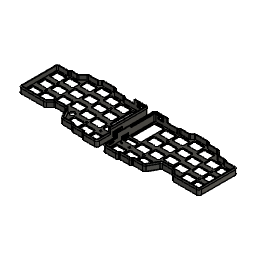
mriya-bumper-mjf-v1.14 (Autodesk Fusion 360 design; units mm, degrees)
Autodesk Fusion 360 part; units mm, degrees
(part 1 of 2)
sketch "mriya-bumper-mjf" plane through (0, 0, 0) normal (0, 0, 1) x (1, 0, 0)
  line L0 (-101.0213, 15.6719) -> (-94.7787, 21.9145) construction
  line L1 (-26.4858, 1.079) -> (-27.6142, 2.2074) construction
  line L2 (-138.1, 14.7932) -> (-103.1426, 14.7932) construction
  line L3 (-44.0716, 2.7932) -> (-29.0284, 2.7932) construction
  line L4 (-8.6, 0.4932) -> (-25.0716, 0.4932) construction
  line L5 (-64.4741, 6.1094) -> (-72.7517, 20.7608) construction
  line L6 (-45.4858, 3.379) -> (-46.6142, 4.5074) construction
  line L7 (-122.6142, 71.579) -> (-121.4858, 72.7074) construction
  line L8 (-101.0716, 81.2932) -> (-87.2284, 81.2932) construction
  line L9 (-138.1, 70.9932) -> (-124.0284, 70.9932) construction
  line L10 (-92.6574, 22.7932) -> (-76.2344, 22.7932) construction
  line L11 (-48.0284, 5.0932) -> (-62.7328, 5.0932) construction
  line L12 (-82.0716, 84.7932) -> (-64.7284, 84.7932) construction
  line L13 (-58.5716, 80.2932) -> (-45.7284, 80.2932) construction
  line L14 (-24.8, 19.4932) -> (-7.1, 19.4932) construction
  line L15 (-25.6, 20.2932) -> (-25.6, 77.9932) construction
  line L16 (-83.4858, 84.2074) -> (-85.8142, 81.879) construction
  line L17 (-63.3142, 84.2074) -> (-59.9858, 80.879) construction
  line L18 (-139.6, 69.4932) -> (-139.6, 16.2932) construction
  line L19 (-43.1858, 78.579) -> (-44.3142, 79.7074) construction
  line L20 (-99.4, 40.3932) -> (-99.4, 27.9932) construction
  line L21 (-98.6, 41.1932) -> (-86.2, 41.1932) construction
  line L22 (-98.6, 27.1932) -> (-86.2, 27.1932) construction
  line L23 (-85.4, 40.3932) -> (-85.4, 27.9932) construction
  line L24 (-42.4, 56.0932) -> (-42.4, 43.6932) construction
  line L25 (-41.6, 56.8932) -> (-29.2, 56.8932) construction
  line L26 (-41.6, 42.8932) -> (-29.2, 42.8932) construction
  line L27 (-28.4, 56.0932) -> (-28.4, 43.6932) construction
  line L28 (-61.4, 58.3932) -> (-61.4, 45.9932) construction
  line L29 (-60.6, 59.1932) -> (-48.2, 59.1932) construction
  line L30 (-60.6, 45.1932) -> (-48.2, 45.1932) construction
  line L31 (-47.4, 58.3932) -> (-47.4, 45.9932) construction
  line L32 (-137.4, 68.0932) -> (-137.4, 55.6932) construction
  line L33 (-136.6, 68.8932) -> (-124.2, 68.8932) construction
  line L34 (-136.6, 54.8932) -> (-124.2, 54.8932) construction
  line L35 (-123.4, 68.0932) -> (-123.4, 55.6932) construction
  line L36 (-61.4, 39.3932) -> (-61.4, 26.9932) construction
  line L37 (-60.6, 40.1932) -> (-48.2, 40.1932) construction
  line L38 (-60.6, 26.1932) -> (-48.2, 26.1932) construction
  line L39 (-47.4, 39.3932) -> (-47.4, 26.9932) construction
  line L40 (-42.4, 18.0932) -> (-42.4, 5.6932) construction
  line L41 (-41.6, 18.8932) -> (-29.2, 18.8932) construction
  line L42 (-41.6, 4.8932) -> (-29.2, 4.8932) construction
  line L43 (-28.4, 18.0932) -> (-28.4, 5.6932) construction
  line L44 (-23.4, 15.7932) -> (-23.4, 3.3932) construction
  line L45 (-22.6, 16.5932) -> (-10.2, 16.5932) construction
  line L46 (-22.6, 2.5932) -> (-10.2, 2.5932) construction
  line L47 (-9.4, 15.7932) -> (-9.4, 3.3932) construction
  line L48 (-137.4, 49.0932) -> (-137.4, 36.6932) construction
  line L49 (-136.6, 49.8932) -> (-124.2, 49.8932) construction
  line L50 (-136.6, 35.8932) -> (-124.2, 35.8932) construction
  line L51 (-123.4, 49.0932) -> (-123.4, 36.6932) construction
  line L52 (-118.4, 51.3932) -> (-118.4, 38.9932) construction
  line L53 (-117.6, 52.1932) -> (-105.2, 52.1932) construction
  line L54 (-117.6, 38.1932) -> (-105.2, 38.1932) construction
  line L55 (-104.4, 51.3932) -> (-104.4, 38.9932) construction
  line L56 (-137.4, 30.0932) -> (-137.4, 17.6932) construction
  line L57 (-136.6, 30.8932) -> (-124.2, 30.8932) construction
  line L58 (-136.6, 16.8932) -> (-124.2, 16.8932) construction
  line L59 (-123.4, 30.0932) -> (-123.4, 17.6932) construction
  line L60 (-61.4, 20.3932) -> (-61.4, 7.9932) construction
  line L61 (-60.6, 21.1932) -> (-48.2, 21.1932) construction
  line L62 (-60.6, 7.1932) -> (-48.2, 7.1932) construction
  line L63 (-47.4, 20.3932) -> (-47.4, 7.9932) construction
  line L64 (-80.4, 43.8932) -> (-80.4, 31.4932) construction
  line L65 (-79.6, 44.6932) -> (-67.2, 44.6932) construction
  line L66 (-79.6, 30.6932) -> (-67.2, 30.6932) construction
  line L67 (-66.4, 43.8932) -> (-66.4, 31.4932) construction
  line L68 (-80.4, 81.8932) -> (-80.4, 69.4932) construction
  line L69 (-79.6, 82.6932) -> (-67.2, 82.6932) construction
  line L70 (-79.6, 68.6932) -> (-67.2, 68.6932) construction
  line L71 (-66.4, 81.8932) -> (-66.4, 69.4932) construction
  line L72 (-42.4, 37.0932) -> (-42.4, 24.6932) construction
  line L73 (-41.6, 37.8932) -> (-29.2, 37.8932) construction
  line L74 (-41.6, 23.8932) -> (-29.2, 23.8932) construction
  line L75 (-28.4, 37.0932) -> (-28.4, 24.6932) construction
  line L76 (-118.4, 32.3932) -> (-118.4, 19.9932) construction
  line L77 (-117.6, 33.1932) -> (-105.2, 33.1932) construction
  line L78 (-117.6, 19.1932) -> (-105.2, 19.1932) construction
  line L79 (-104.4, 32.3932) -> (-104.4, 19.9932) construction
  line L80 (-61.4, 77.3932) -> (-61.4, 64.9932) construction
  line L81 (-60.6, 78.1932) -> (-48.2, 78.1932) construction
  line L82 (-60.6, 64.1932) -> (-48.2, 64.1932) construction
  line L83 (-47.4, 77.3932) -> (-47.4, 64.9932) construction
  line L84 (-42.4, 75.0932) -> (-42.4, 62.6932) construction
  line L85 (-41.6, 75.8932) -> (-29.2, 75.8932) construction
  line L86 (-41.6, 61.8932) -> (-29.2, 61.8932) construction
  line L87 (-28.4, 75.0932) -> (-28.4, 62.6932) construction
  line L88 (-118.4, 70.3932) -> (-118.4, 57.9932) construction
  line L89 (-117.6, 71.1932) -> (-105.2, 71.1932) construction
  line L90 (-117.6, 57.1932) -> (-105.2, 57.1932) construction
  line L91 (-104.4, 70.3932) -> (-104.4, 57.9932) construction
  line L92 (-99.4, 59.3932) -> (-99.4, 46.9932) construction
  line L93 (-98.6, 60.1932) -> (-86.2, 60.1932) construction
  line L94 (-98.6, 46.1932) -> (-86.2, 46.1932) construction
  line L95 (-85.4, 59.3932) -> (-85.4, 46.9932) construction
  line L96 (-80.4, 62.8932) -> (-80.4, 50.4932) construction
  line L97 (-79.6, 63.6932) -> (-67.2, 63.6932) construction
  line L98 (-79.6, 49.6932) -> (-67.2, 49.6932) construction
  line L99 (-66.4, 62.8932) -> (-66.4, 50.4932) construction
  line L100 (-99.4, 78.3932) -> (-99.4, 65.9932) construction
  line L101 (-98.6, 79.1932) -> (-86.2, 79.1932) construction
  line L102 (-98.6, 65.1932) -> (-86.2, 65.1932) construction
  line L103 (-85.4, 78.3932) -> (-85.4, 65.9932) construction
  circle A0 centre (-120.9, 53.5432) radius 1.7
  circle A1 centre (-120.9, 34.5432) radius 1.7
  circle A2 centre (-68.5, 23.5932) radius 4
  circle A3 centre (-44.9, 22.5432) radius 1.7
  circle A4 centre (-44.9, 60.5432) radius 1.7
  arc A5 (-43.1858, 78.579) -> (-41.7716, 77.9932) centre (-41.7716, 79.9932) ccw construction
  arc A6 (-44.3142, 79.7074) -> (-45.7284, 80.2932) centre (-45.7285, 78.2931) ccw construction
  arc A7 (-59.9858, 80.879) -> (-58.5716, 80.2932) centre (-58.5716, 82.2931) ccw construction
  arc A8 (-63.3142, 84.2074) -> (-64.7284, 84.7932) centre (-64.7285, 82.7931) ccw construction
  arc A9 (-82.0716, 84.7932) -> (-83.4858, 84.2074) centre (-82.0716, 82.7933) ccw construction
  arc A10 (-87.2284, 81.2932) -> (-85.8142, 81.879) centre (-87.2284, 83.2932) ccw construction
  arc A11 (-101.0716, 81.2932) -> (-102.4858, 80.7074) centre (-101.0716, 79.2933) ccw construction
  arc A12 (-120.0716, 73.2932) -> (-121.4858, 72.7074) centre (-120.0716, 71.2933) ccw construction
  arc A13 (-124.0284, 70.9932) -> (-122.6142, 71.579) centre (-124.0284, 72.9932) ccw construction
  arc A14 (-138.1, 70.9932) -> (-139.6, 69.4932) centre (-138.1, 69.4932) ccw construction
  arc A15 (-139.6, 16.2932) -> (-138.1, 14.7932) centre (-138.1, 16.2932) ccw construction
  arc A16 (-103.1426, 14.7932) -> (-101.0213, 15.6719) centre (-103.1426, 17.7931) ccw construction
  arc A17 (-92.6574, 22.7932) -> (-94.7787, 21.9145) centre (-92.6573, 19.7931) ccw construction
  arc A18 (-72.7517, 20.7608) -> (-76.2344, 22.7932) centre (-76.2344, 18.793) ccw construction
  arc A19 (-64.4741, 6.1094) -> (-62.7328, 5.0932) centre (-62.7328, 7.0932) ccw construction
  arc A20 (-46.6142, 4.5074) -> (-48.0284, 5.0932) centre (-48.0284, 3.0933) ccw construction
  arc A21 (-45.4858, 3.379) -> (-44.0716, 2.7932) centre (-44.0715, 4.7933) ccw construction
  arc A22 (-27.6142, 2.2074) -> (-29.0284, 2.7932) centre (-29.0284, 0.7933) ccw construction
  arc A23 (-26.4858, 1.079) -> (-25.0716, 0.4932) centre (-25.0715, 2.4933) ccw construction
  arc A24 (-8.6, 0.4932) -> (-7.1, 1.9932) centre (-8.6, 1.9932) ccw construction
  line L104 (-7.1, 1.9932) -> (-7.1, 76.4932) construction
  line L105 (-41.7716, 77.9932) -> (-8.6, 77.9932) construction
  arc A25 (-7.1, 76.4932) -> (-8.6, 77.9932) centre (-8.6, 76.4932) ccw construction
  arc A26 (-136.6, 68.8932) -> (-137.4, 68.0932) centre (-136.6, 68.0932) ccw construction
  arc A27 (-123.4, 68.0932) -> (-124.2, 68.8932) centre (-124.2, 68.0932) ccw construction
  arc A28 (-124.2, 54.8932) -> (-123.4, 55.6932) centre (-124.2, 55.6932) ccw construction
  arc A29 (-137.4, 55.6932) -> (-136.6, 54.8932) centre (-136.6, 55.6932) ccw construction
  arc A30 (-136.6, 49.8932) -> (-137.4, 49.0932) centre (-136.6, 49.0932) ccw construction
  arc A31 (-123.4, 49.0932) -> (-124.2, 49.8932) centre (-124.2, 49.0932) ccw construction
  arc A32 (-124.2, 35.8932) -> (-123.4, 36.6932) centre (-124.2, 36.6932) ccw construction
  arc A33 (-137.4, 36.6932) -> (-136.6, 35.8932) centre (-136.6, 36.6932) ccw construction
  arc A34 (-136.6, 30.8932) -> (-137.4, 30.0932) centre (-136.6, 30.0932) ccw construction
  arc A35 (-123.4, 30.0932) -> (-124.2, 30.8932) centre (-124.2, 30.0932) ccw construction
  arc A36 (-124.2, 16.8932) -> (-123.4, 17.6932) centre (-124.2, 17.6932) ccw construction
  arc A37 (-137.4, 17.6932) -> (-136.6, 16.8932) centre (-136.6, 17.6932) ccw construction
  arc A38 (-118.4, 19.9932) -> (-117.6, 19.1932) centre (-117.6, 19.9932) ccw construction
  arc A39 (-105.2, 19.1932) -> (-104.4, 19.9932) centre (-105.2, 19.9932) ccw construction
  arc A40 (-104.4, 32.3932) -> (-105.2, 33.1932) centre (-105.2, 32.3932) ccw construction
  arc A41 (-117.6, 33.1932) -> (-118.4, 32.3932) centre (-117.6, 32.3932) ccw construction
  arc A42 (-105.2, 38.1932) -> (-104.4, 38.9932) centre (-105.2, 38.9932) ccw construction
  arc A43 (-118.4, 38.9932) -> (-117.6, 38.1932) centre (-117.6, 38.9932) ccw construction
  arc A44 (-117.6, 52.1932) -> (-118.4, 51.3932) centre (-117.6, 51.3932) ccw construction
  arc A45 (-104.4, 51.3932) -> (-105.2, 52.1932) centre (-105.2, 51.3932) ccw construction
  arc A46 (-118.4, 57.9932) -> (-117.6, 57.1932) centre (-117.6, 57.9932) ccw construction
  arc A47 (-105.2, 57.1932) -> (-104.4, 57.9932) centre (-105.2, 57.9932) ccw construction
  arc A48 (-104.4, 70.3932) -> (-105.2, 71.1932) centre (-105.2, 70.3932) ccw construction
  arc A49 (-117.6, 71.1932) -> (-118.4, 70.3932) centre (-117.6, 70.3932) ccw construction
  arc A50 (-98.6, 79.1932) -> (-99.4, 78.3932) centre (-98.6, 78.3932) ccw construction
  arc A51 (-85.4, 78.3932) -> (-86.2, 79.1932) centre (-86.2, 78.3932) ccw construction
  arc A52 (-86.2, 65.1932) -> (-85.4, 65.9932) centre (-86.2, 65.9932) ccw construction
  arc A53 (-99.4, 65.9932) -> (-98.6, 65.1932) centre (-98.6, 65.9932) ccw construction
  arc A54 (-98.6, 60.1932) -> (-99.4, 59.3932) centre (-98.6, 59.3932) ccw construction
  arc A55 (-85.4, 59.3932) -> (-86.2, 60.1932) centre (-86.2, 59.3932) ccw construction
  arc A56 (-86.2, 46.1932) -> (-85.4, 46.9932) centre (-86.2, 46.9932) ccw construction
  arc A57 (-99.4, 46.9932) -> (-98.6, 46.1932) centre (-98.6, 46.9932) ccw construction
  arc A58 (-98.6, 41.1932) -> (-99.4, 40.3932) centre (-98.6, 40.3932) ccw construction
  arc A59 (-99.4, 27.9932) -> (-98.6, 27.1932) centre (-98.6, 27.9932) ccw construction
  arc A60 (-86.2, 27.1932) -> (-85.4, 27.9932) centre (-86.2, 27.9932) ccw construction
  arc A61 (-85.4, 40.3932) -> (-86.2, 41.1932) centre (-86.2, 40.3932) ccw construction
  arc A62 (-80.4, 31.4932) -> (-79.6, 30.6932) centre (-79.6, 31.4932) ccw construction
  arc A63 (-79.6, 44.6932) -> (-80.4, 43.8932) centre (-79.6, 43.8932) ccw construction
  arc A64 (-66.4, 43.8932) -> (-67.2, 44.6932) centre (-67.2, 43.8932) ccw construction
  arc A65 (-67.2, 30.6932) -> (-66.4, 31.4932) centre (-67.2, 31.4932) ccw construction
  arc A66 (-67.2, 49.6932) -> (-66.4, 50.4932) centre (-67.2, 50.4932) ccw construction
  arc A67 (-80.4, 50.4932) -> (-79.6, 49.6932) centre (-79.6, 50.4932) ccw construction
  arc A68 (-79.6, 63.6932) -> (-80.4, 62.8932) centre (-79.6, 62.8932) ccw construction
  arc A69 (-66.4, 62.8932) -> (-67.2, 63.6932) centre (-67.2, 62.8932) ccw construction
  arc A70 (-67.2, 68.6932) -> (-66.4, 69.4932) centre (-67.2, 69.4932) ccw construction
  arc A71 (-80.4, 69.4932) -> (-79.6, 68.6932) centre (-79.6, 69.4932) ccw construction
  arc A72 (-79.6, 82.6932) -> (-80.4, 81.8932) centre (-79.6, 81.8932) ccw construction
  arc A73 (-66.4, 81.8932) -> (-67.2, 82.6932) centre (-67.2, 81.8932) ccw construction
  arc A74 (-60.6, 78.1932) -> (-61.4, 77.3932) centre (-60.6, 77.3932) ccw construction
  arc A75 (-61.4, 64.9932) -> (-60.6, 64.1932) centre (-60.6, 64.9932) ccw construction
  arc A76 (-48.2, 64.1932) -> (-47.4, 64.9932) centre (-48.2, 64.9932) ccw construction
  arc A77 (-47.4, 77.3932) -> (-48.2, 78.1932) centre (-48.2, 77.3932) ccw construction
  arc A78 (-47.4, 58.3932) -> (-48.2, 59.1932) centre (-48.2, 58.3932) ccw construction
  arc A79 (-60.6, 59.1932) -> (-61.4, 58.3932) centre (-60.6, 58.3932) ccw construction
  arc A80 (-61.4, 45.9932) -> (-60.6, 45.1932) centre (-60.6, 45.9932) ccw construction
  arc A81 (-48.2, 45.1932) -> (-47.4, 45.9932) centre (-48.2, 45.9932) ccw construction
  arc A82 (-47.4, 39.3932) -> (-48.2, 40.1932) centre (-48.2, 39.3932) ccw construction
  arc A83 (-60.6, 40.1932) -> (-61.4, 39.3932) centre (-60.6, 39.3932) ccw construction
  arc A84 (-61.4, 26.9932) -> (-60.6, 26.1932) centre (-60.6, 26.9932) ccw construction
  arc A85 (-48.2, 26.1932) -> (-47.4, 26.9932) centre (-48.2, 26.9932) ccw construction
  arc A86 (-47.4, 20.3932) -> (-48.2, 21.1932) centre (-48.2, 20.3932) ccw construction
  arc A87 (-60.6, 21.1932) -> (-61.4, 20.3932) centre (-60.6, 20.3932) ccw construction
  arc A88 (-61.4, 7.9932) -> (-60.6, 7.1932) centre (-60.6, 7.9932) ccw construction
  arc A89 (-48.2, 7.1932) -> (-47.4, 7.9932) centre (-48.2, 7.9932) ccw construction
  arc A90 (-42.4, 5.6932) -> (-41.6, 4.8932) centre (-41.6, 5.6932) ccw construction
  arc A91 (-29.2, 4.8932) -> (-28.4, 5.6932) centre (-29.2, 5.6932) ccw construction
  arc A92 (-28.4, 18.0932) -> (-29.2, 18.8932) centre (-29.2, 18.0932) ccw construction
  arc A93 (-41.6, 18.8932) -> (-42.4, 18.0932) centre (-41.6, 18.0932) ccw construction
  arc A94 (-23.4, 3.3932) -> (-22.6, 2.5932) centre (-22.6, 3.3932) ccw construction
  arc A95 (-10.2, 2.5932) -> (-9.4, 3.3932) centre (-10.2, 3.3932) ccw construction
  arc A96 (-9.4, 15.7932) -> (-10.2, 16.5932) centre (-10.2, 15.7932) ccw construction
  arc A97 (-22.6, 16.5932) -> (-23.4, 15.7932) centre (-22.6, 15.7932) ccw construction
  arc A98 (-29.2, 23.8932) -> (-28.4, 24.6932) centre (-29.2, 24.6932) ccw construction
  arc A99 (-42.4, 24.6932) -> (-41.6, 23.8932) centre (-41.6, 24.6932) ccw construction
  arc A100 (-41.6, 37.8932) -> (-42.4, 37.0932) centre (-41.6, 37.0932) ccw construction
  arc A101 (-28.4, 37.0932) -> (-29.2, 37.8932) centre (-29.2, 37.0932) ccw construction
  arc A102 (-29.2, 42.8932) -> (-28.4, 43.6932) centre (-29.2, 43.6932) ccw construction
  arc A103 (-42.4, 43.6932) -> (-41.6, 42.8932) centre (-41.6, 43.6932) ccw construction
  arc A104 (-41.6, 56.8932) -> (-42.4, 56.0932) centre (-41.6, 56.0932) ccw construction
  arc A105 (-28.4, 56.0932) -> (-29.2, 56.8932) centre (-29.2, 56.0932) ccw construction
  arc A106 (-29.2, 61.8932) -> (-28.4, 62.6932) centre (-29.2, 62.6932) ccw construction
  arc A107 (-42.4, 62.6932) -> (-41.6, 61.8932) centre (-41.6, 62.6932) ccw construction
  arc A108 (-41.6, 75.8932) -> (-42.4, 75.0932) centre (-41.6, 75.0932) ccw construction
  arc A109 (-28.4, 75.0932) -> (-29.2, 75.8932) centre (-29.2, 75.0932) ccw construction
  circle A110 centre (-22.6, 22.4932) radius 1.1
  circle A111 centre (-10.1, 22.4932) radius 1.1
  line L106 (-7, 19.2932) -> (-4.5, 19.2932)
  line L107 (-25.8, 78.0932) -> (-25.8, 80.5932)
  line L108 (-20.5, 77.4932) -> (-8.6, 77.4932)
  line L109 (-7.6, 40.5932) -> (-7.6, 76.4932)
  line L110 (-7.6, 12.9932) -> (-7.6, 6.1932)
  line L111 (-102.4858, 80.7074) -> (-109.0213, 74.1719) construction
  line L112 (-120.0716, 73.2932) -> (-111.1426, 73.2932) construction
  arc A112 (-111.1426, 73.2932) -> (-109.0213, 74.1719) centre (-111.1426, 76.2932) ccw construction
  arc A113 (-64.7284, 82.7932) -> (-64.7285, 82.7932) centre (-64.7285, 82.7931) ccw
  arc A114 (-45.7284, 78.2932) -> (-45.7285, 78.2932) centre (-45.7285, 78.2931) ccw
  arc A115 (-25.0716, 2.4932) -> (-25.0715, 2.4932) centre (-25.0715, 2.4933) ccw
  arc A116 (-44.0716, 4.7932) -> (-44.0715, 4.7932) centre (-44.0715, 4.7933) ccw
  line L113 (-138.9, 58.3932) -> (-138.9, 66.8932)
  line L114 (-136.9, 68.8932) -> (-123.9, 68.8932)
  arc A117 (-121.9, 66.8932) -> (-123.9, 68.8932) centre (-123.9, 66.8932) ccw
  arc A118 (-136.9, 68.8932) -> (-138.9, 66.8932) centre (-136.9, 66.8932) ccw
  line L115 (-104.9, 58.6932) -> (-117.9, 58.6932)
  line L116 (-119.9, 60.6932) -> (-119.9, 69.1932)
  arc A119 (-117.9, 71.1932) -> (-119.9, 69.1932) centre (-117.9, 69.1932) ccw
  line L117 (-117.9, 71.1932) -> (-104.9, 71.1932)
  arc A120 (-102.9, 69.1932) -> (-104.9, 71.1932) centre (-104.9, 69.1932) ccw
  line L118 (-102.9, 69.1932) -> (-102.9, 60.6932)
  line L119 (-85.9, 66.6932) -> (-98.9, 66.6932)
  line L120 (-100.9, 68.6932) -> (-100.9, 77.1932)
  arc A121 (-98.9, 79.1932) -> (-100.9, 77.1932) centre (-98.9, 77.1932) ccw
  line L121 (-98.9, 79.1932) -> (-85.9, 79.1932)
  arc A122 (-83.9, 77.1932) -> (-85.9, 79.1932) centre (-85.9, 77.1932) ccw
  line L122 (-83.9, 77.1932) -> (-83.9, 68.6932)
  line L123 (-66.9, 70.1932) -> (-79.9, 70.1932)
  line L124 (-81.9, 72.1932) -> (-81.9, 80.6932)
  arc A123 (-79.9, 82.6932) -> (-81.9, 80.6932) centre (-79.9, 80.6932) ccw
  line L125 (-79.9, 82.6932) -> (-66.9, 82.6932)
  arc A124 (-64.9, 80.6932) -> (-66.9, 82.6932) centre (-66.9, 80.6932) ccw
  line L126 (-64.9, 80.6932) -> (-64.9, 72.1932)
  line L127 (-47.9, 65.6932) -> (-60.9, 65.6932)
  line L128 (-62.9, 67.6932) -> (-62.9, 76.1932)
  arc A125 (-60.9, 78.1932) -> (-62.9, 76.1932) centre (-60.9, 76.1932) ccw
  line L129 (-60.9, 78.1932) -> (-47.9, 78.1932)
  arc A126 (-45.9, 76.1932) -> (-47.9, 78.1932) centre (-47.9, 76.1932) ccw
  line L130 (-45.9, 76.1932) -> (-45.9, 67.6932)
  line L131 (-43.9, 65.3932) -> (-43.9, 73.8932)
  arc A127 (-41.9, 75.8932) -> (-43.9, 73.8932) centre (-41.9, 73.8932) ccw
  line L132 (-41.9, 75.8932) -> (-28.9, 75.8932)
  arc A128 (-26.9, 73.8932) -> (-28.9, 75.8932) centre (-28.9, 73.8932) ccw
  line L133 (-26.9, 73.8932) -> (-26.9, 65.3932)
  arc A129 (-9.9, 26.8932) -> (-7.9, 28.8932) centre (-9.9, 28.8932) ccw
  line L134 (-9.9, 26.8932) -> (-22.9, 26.8932)
  arc A130 (-24.9, 28.8932) -> (-22.9, 26.8932) centre (-22.9, 28.8932) ccw
  arc A131 (-22.9, 75.8932) -> (-24.9, 73.8932) centre (-22.9, 73.8932) ccw
  arc A132 (-7.9, 73.8932) -> (-9.9, 75.8932) centre (-9.9, 73.8932) ccw
  line L135 (-28.9, 63.3932) -> (-41.9, 63.3932)
  line L136 (-121.9, 66.8932) -> (-121.9, 58.3932)
  line L137 (-123.9, 56.3932) -> (-136.9, 56.3932)
  line L138 (-122.6849, 71.6497) -> (-121.5565, 72.7781)
  arc A133 (-120.0716, 73.3932) -> (-121.5565, 72.7781) centre (-120.0716, 71.2933) ccw
  line L139 (-120.0716, 73.3932) -> (-111.1426, 73.3932)
  arc A134 (-111.1426, 73.3932) -> (-109.092, 74.2426) centre (-111.1426, 76.2932) ccw
  line L140 (-102.5565, 80.7781) -> (-109.092, 74.2426)
  arc A135 (-101.0716, 81.3932) -> (-102.5565, 80.7781) centre (-101.0716, 79.2933) ccw
  line L141 (-101.0716, 81.3932) -> (-87.2284, 81.3932)
  arc A136 (-87.2284, 81.3932) -> (-85.8849, 81.9497) centre (-87.2284, 83.2932) ccw
  line L142 (-83.5565, 84.2781) -> (-85.8849, 81.9497)
  arc A137 (-82.0716, 84.8932) -> (-83.5565, 84.2781) centre (-82.0716, 82.7933) ccw
  line L143 (-82.0716, 84.8932) -> (-64.7284, 84.8932)
  arc A138 (-63.2435, 84.2781) -> (-64.7284, 84.8932) centre (-64.7285, 82.7931) ccw
  line L144 (-63.2435, 84.2781) -> (-59.9151, 80.9497)
  arc A139 (-59.9151, 80.9497) -> (-58.5716, 80.3932) centre (-58.5716, 82.2931) ccw
  line L145 (-58.5716, 80.3932) -> (-45.7284, 80.3932)
  arc A140 (-44.2435, 79.7781) -> (-45.7284, 80.3932) centre (-45.7285, 78.2931) ccw
  line L146 (-43.1151, 78.6497) -> (-44.2435, 79.7781)
  arc A141 (-43.1151, 78.6497) -> (-41.7716, 78.0932) centre (-41.7716, 79.9932) ccw
  line L147 (-41.7716, 78.0932) -> (-8.6, 78.0932)
  arc A142 (-7, 76.4932) -> (-8.6, 78.0932) centre (-8.6, 76.4932) ccw
  line L148 (-7, 1.9932) -> (-7, 76.4932)
  arc A143 (-8.6, 0.3932) -> (-7, 1.9932) centre (-8.6, 1.9932) ccw
  line L149 (-8.6, 0.3932) -> (-25.0716, 0.3932)
  arc A144 (-26.5565, 1.0083) -> (-25.0716, 0.3932) centre (-25.0715, 2.4933) ccw
  line L150 (-26.5565, 1.0083) -> (-27.6849, 2.1367)
  arc A145 (-27.6849, 2.1367) -> (-29.0284, 2.6932) centre (-29.0284, 0.7933) ccw
  line L151 (-44.0716, 2.6932) -> (-29.0284, 2.6932)
  arc A146 (-45.5565, 3.3083) -> (-44.0716, 2.6932) centre (-44.0715, 4.7933) ccw
  line L152 (-45.5565, 3.3083) -> (-46.6849, 4.4367)
  arc A147 (-46.6849, 4.4367) -> (-48.0284, 4.9932) centre (-48.0284, 3.0933) ccw
  line L153 (-48.0284, 4.9932) -> (-62.7328, 4.9932)
  arc A148 (-64.5612, 6.0602) -> (-62.7328, 4.9932) centre (-62.7328, 7.0932) ccw
  line L154 (-64.5612, 6.0602) -> (-72.8388, 20.7116)
  arc A149 (-72.8388, 20.7116) -> (-76.2344, 22.6932) centre (-76.2344, 18.793) ccw
  line L155 (-92.6574, 22.6932) -> (-76.2344, 22.6932)
  arc A150 (-92.6574, 22.6932) -> (-94.708, 21.8438) centre (-92.6573, 19.7931) ccw
  line L156 (-100.9506, 15.6012) -> (-94.708, 21.8438)
  arc A151 (-103.1426, 14.6932) -> (-100.9506, 15.6012) centre (-103.1426, 17.7931) ccw
  line L157 (-138.1, 14.6932) -> (-103.1426, 14.6932)
  arc A152 (-139.7, 16.2932) -> (-138.1, 14.6932) centre (-138.1, 16.2932) ccw
  line L158 (-139.7, 69.4932) -> (-139.7, 16.2932)
  arc A153 (-138.1, 71.0932) -> (-139.7, 69.4932) centre (-138.1, 69.4932) ccw
  line L159 (-138.1, 71.0932) -> (-124.0284, 71.0932)
  arc A154 (-124.0284, 71.0932) -> (-122.6849, 71.6497) centre (-124.0284, 72.9932) ccw
  line L160 (-120.3201, 75.8932) -> (-111.5983, 75.8932)
  line L161 (-101.3201, 83.8932) -> (-88.0983, 83.8932)
  line L162 (-82.3201, 87.3932) -> (-64.4799, 87.3932)
  line L163 (-57.7017, 82.8932) -> (-45.4799, 82.8932)
  line L164 (-40.9017, 80.5932) -> (-8.5, 80.5932)
  line L165 (-4.5, 1.8932) -> (-4.5, 76.5932)
  line L166 (-8.5, -2.1068) -> (-25.3201, -2.1068)
  line L167 (-44.3201, 0.1932) -> (-29.8983, 0.1932)
  line L168 (-48.8983, 2.4932) -> (-63.083, 2.4932)
  line L169 (-91.9946, 20.1932) -> (-77.1681, 20.1932)
  line L170 (-138.2, 12.1932) -> (-102.687, 12.1932)
  line L171 (-142.2, 69.5932) -> (-142.2, 16.1932)
  line L172 (-138.2, 73.5932) -> (-124.8983, 73.5932)
  line L173 (-66.5656, 4.5256) -> (-74.5561, 18.6689)
  line L174 (-99.505, 13.5112) -> (-93.4088, 19.6074)
  arc A155 (-138.2, 73.5932) -> (-142.2, 69.5932) centre (-138.2, 69.5932) ccw
  arc A156 (-142.2, 16.1932) -> (-138.2, 12.1932) centre (-138.2, 16.1932) ccw
  arc A157 (-8.5, -2.1068) -> (-4.5, 1.8932) centre (-8.5, 1.8932) ccw
  arc A158 (-4.5, 76.5932) -> (-8.5, 80.5932) centre (-8.5, 76.5932) ccw
  arc A159 (-111.5983, 75.8932) -> (-110.5376, 76.3325) centre (-111.5983, 77.3932) ccw
  arc A160 (-66.5656, 4.5256) -> (-63.083, 2.4932) centre (-63.083, 6.4932) ccw
  arc A161 (-74.5561, 18.6689) -> (-77.1681, 20.1932) centre (-77.1681, 17.1932) ccw
  arc A162 (-91.9946, 20.1932) -> (-93.4088, 19.6074) centre (-91.9946, 18.1932) ccw
  arc A163 (-102.687, 12.1932) -> (-99.505, 13.5112) centre (-102.687, 16.6932) ccw
  line L175 (-22.9, 34.8932) -> (-9.9, 34.8932)
  line L176 (-24.9, 28.8932) -> (-24.9, 32.8932)
  line L177 (-24.9, 39.8932) -> (-24.9, 73.8932)
  line L178 (-7.9, 73.8932) -> (-7.9, 39.8932)
  line L179 (-7.9, 32.8932) -> (-7.9, 28.8932)
  arc A164 (-24.9, 39.8932) -> (-22.9, 37.8932) centre (-22.9, 39.8932) ccw
  arc A165 (-9.9, 37.8932) -> (-7.9, 39.8932) centre (-9.9, 39.8932) ccw
  arc A166 (-22.9, 34.8932) -> (-24.9, 32.8932) centre (-22.9, 32.8932) ccw
  arc A167 (-7.9, 32.8932) -> (-9.9, 34.8932) centre (-9.9, 32.8932) ccw
  line L180 (-123.8376, 74.0325) -> (-123.1485, 74.7216)
  line L181 (-110.5376, 76.3325) -> (-104.1485, 82.7216)
  line L182 (-87.0376, 84.3325) -> (-85.1485, 86.2216)
  line L183 (-61.6515, 86.2216) -> (-58.7624, 83.3325)
  line L184 (-42.6515, 81.7216) -> (-41.9624, 81.0325)
  line L185 (-28.1485, -0.9352) -> (-28.8376, -0.2461)
  line L186 (-47.8376, 2.0539) -> (-47.1485, 1.3648)
  arc A168 (-47.8376, 2.0539) -> (-48.8983, 2.4932) centre (-48.8983, 0.9932) ccw
  arc A169 (-28.8376, -0.2461) -> (-29.8983, 0.1932) centre (-29.8983, -1.3068) ccw
  arc A170 (-47.1485, 1.3648) -> (-44.3201, 0.1932) centre (-44.3201, 4.1932) ccw
  arc A171 (-28.1485, -0.9352) -> (-25.3201, -2.1068) centre (-25.3201, 1.8932) ccw
  arc A172 (-41.9624, 81.0325) -> (-40.9017, 80.5932) centre (-40.9017, 82.0932) ccw
  arc A173 (-42.6515, 81.7216) -> (-45.4799, 82.8932) centre (-45.4799, 78.8932) ccw
  arc A174 (-82.3201, 87.3932) -> (-85.1485, 86.2216) centre (-82.3201, 83.3932) ccw
  arc A175 (-61.6515, 86.2216) -> (-64.4799, 87.3932) centre (-64.4799, 83.3932) ccw
  arc A176 (-58.7624, 83.3325) -> (-57.7017, 82.8932) centre (-57.7017, 84.3932) ccw
  arc A177 (-88.0983, 83.8932) -> (-87.0376, 84.3325) centre (-88.0983, 85.3932) ccw
  arc A178 (-101.3201, 83.8932) -> (-104.1485, 82.7216) centre (-101.3201, 79.8932) ccw
  arc A179 (-120.3201, 75.8932) -> (-123.1485, 74.7216) centre (-120.3201, 71.8932) ccw
  arc A180 (-124.8983, 73.5932) -> (-123.8376, 74.0325) centre (-124.8983, 75.0932) ccw
  circle A181 centre (-22.6, 22.4932) radius 2.1
  circle A182 centre (-10.1, 22.4932) radius 2.1
  arc A183 (-7.6, 6.1932) -> (-7, 5.5932) centre (-7, 6.1932) ccw
  arc A184 (-7, 13.5932) -> (-7.6, 12.9932) centre (-7, 12.9932) ccw
  arc A185 (-21.1, 78.0932) -> (-20.5, 77.4932) centre (-20.5, 78.0932) ccw
  arc A186 (-7.6, 76.4932) -> (-8.6, 77.4932) centre (-8.6, 76.4932) ccw
  arc A187 (-25.6, 20.2932) -> (-24.8, 19.4932) centre (-24.8, 20.2932) ccw construction
  arc A188 (-138.9, 58.3932) -> (-136.9, 56.3932) centre (-136.9, 58.3932) ccw
  arc A189 (-123.9, 56.3932) -> (-121.9, 58.3932) centre (-123.9, 58.3932) ccw
  arc A190 (-119.9, 60.6932) -> (-117.9, 58.6932) centre (-117.9, 60.6932) ccw
  arc A191 (-104.9, 58.6932) -> (-102.9, 60.6932) centre (-104.9, 60.6932) ccw
  arc A192 (-100.9, 68.6932) -> (-98.9, 66.6932) centre (-98.9, 68.6932) ccw
  arc A193 (-85.9, 66.6932) -> (-83.9, 68.6932) centre (-85.9, 68.6932) ccw
  arc A194 (-81.9, 72.1932) -> (-79.9, 70.1932) centre (-79.9, 72.1932) ccw
  arc A195 (-66.9, 70.1932) -> (-64.9, 72.1932) centre (-66.9, 72.1932) ccw
  arc A196 (-62.9, 67.6932) -> (-60.9, 65.6932) centre (-60.9, 67.6932) ccw
  arc A197 (-47.9, 65.6932) -> (-45.9, 67.6932) centre (-47.9, 67.6932) ccw
  arc A198 (-43.9, 65.3932) -> (-41.9, 63.3932) centre (-41.9, 65.3932) ccw
  arc A199 (-28.9, 63.3932) -> (-26.9, 65.3932) centre (-28.9, 65.3932) ccw
  line L187 (-121.9, 47.8932) -> (-121.9, 39.3932)
  arc A200 (-121.9, 47.8932) -> (-123.9, 49.8932) centre (-123.9, 47.8932) ccw
  line L188 (-136.9, 49.8932) -> (-123.9, 49.8932)
  arc A201 (-136.9, 49.8932) -> (-138.9, 47.8932) centre (-136.9, 47.8932) ccw
  line L189 (-138.9, 39.3932) -> (-138.9, 47.8932)
  arc A202 (-138.9, 39.3932) -> (-136.9, 37.3932) centre (-136.9, 39.3932) ccw
  line L190 (-123.9, 37.3932) -> (-136.9, 37.3932)
  arc A203 (-123.9, 37.3932) -> (-121.9, 39.3932) centre (-123.9, 39.3932) ccw
  arc A204 (-104.9, 39.6932) -> (-102.9, 41.6932) centre (-104.9, 41.6932) ccw
  line L191 (-104.9, 39.6932) -> (-117.9, 39.6932)
  arc A205 (-119.9, 41.6932) -> (-117.9, 39.6932) centre (-117.9, 41.6932) ccw
  line L192 (-119.9, 41.6932) -> (-119.9, 49.7719)
  line L193 (-117.4787, 52.1932) -> (-104.9, 52.1932)
  arc A206 (-102.9, 50.1932) -> (-104.9, 52.1932) centre (-104.9, 50.1932) ccw
  line L194 (-102.9, 50.1932) -> (-102.9, 41.6932)
  arc A207 (-85.9, 47.6932) -> (-83.9, 49.6932) centre (-85.9, 49.6932) ccw
  line L195 (-85.9, 47.6932) -> (-98.9, 47.6932)
  arc A208 (-100.9, 49.6932) -> (-98.9, 47.6932) centre (-98.9, 49.6932) ccw
  line L196 (-100.9, 49.6932) -> (-100.9, 58.1932)
  arc A209 (-98.9, 60.1932) -> (-100.9, 58.1932) centre (-98.9, 58.1932) ccw
  line L197 (-98.9, 60.1932) -> (-85.9, 60.1932)
  arc A210 (-83.9, 58.1932) -> (-85.9, 60.1932) centre (-85.9, 58.1932) ccw
  line L198 (-83.9, 58.1932) -> (-83.9, 49.6932)
  arc A211 (-79.9, 63.6932) -> (-81.9, 61.6932) centre (-79.9, 61.6932) ccw
  line L199 (-79.9, 63.6932) -> (-66.9, 63.6932)
  arc A212 (-64.9, 61.6932) -> (-66.9, 63.6932) centre (-66.9, 61.6932) ccw
  line L200 (-64.9, 61.6932) -> (-64.9, 53.1932)
  arc A213 (-66.9, 51.1932) -> (-64.9, 53.1932) centre (-66.9, 53.1932) ccw
  line L201 (-66.9, 51.1932) -> (-79.9, 51.1932)
  arc A214 (-81.9, 53.1932) -> (-79.9, 51.1932) centre (-79.9, 53.1932) ccw
  line L202 (-81.9, 53.1932) -> (-81.9, 61.6932)
  arc A215 (-60.9, 59.1932) -> (-62.9, 57.1932) centre (-60.9, 57.1932) ccw
  line L203 (-60.9, 59.1932) -> (-48.3213, 59.1932)
  line L204 (-45.9, 56.7719) -> (-45.9, 48.6932)
  arc A216 (-47.9, 46.6932) -> (-45.9, 48.6932) centre (-47.9, 48.6932) ccw
  line L205 (-47.9, 46.6932) -> (-60.9, 46.6932)
  arc A217 (-62.9, 48.6932) -> (-60.9, 46.6932) centre (-60.9, 48.6932) ccw
  line L206 (-62.9, 48.6932) -> (-62.9, 57.1932)
  arc A218 (-41.9, 56.8932) -> (-43.9, 54.8932) centre (-41.9, 54.8932) ccw
  line L207 (-41.9, 56.8932) -> (-28.9, 56.8932)
  arc A219 (-26.9, 54.8932) -> (-28.9, 56.8932) centre (-28.9, 54.8932) ccw
  line L208 (-26.9, 54.8932) -> (-26.9, 46.3932)
  arc A220 (-28.9, 44.3932) -> (-26.9, 46.3932) centre (-28.9, 46.3932) ccw
  line L209 (-28.9, 44.3932) -> (-41.9, 44.3932)
  arc A221 (-43.9, 46.3932) -> (-41.9, 44.3932) centre (-41.9, 46.3932) ccw
  line L210 (-43.9, 46.3932) -> (-43.9, 54.8932)
  arc A222 (-123.9, 18.3932) -> (-121.9, 20.3932) centre (-123.9, 20.3932) ccw
  line L211 (-123.9, 18.3932) -> (-136.9, 18.3932)
  arc A223 (-138.9, 20.3932) -> (-136.9, 18.3932) centre (-136.9, 20.3932) ccw
  line L212 (-138.9, 20.3932) -> (-138.9, 28.8932)
  arc A224 (-136.9, 30.8932) -> (-138.9, 28.8932) centre (-136.9, 28.8932) ccw
  line L213 (-136.9, 30.8932) -> (-123.9, 30.8932)
  arc A225 (-121.9, 28.8932) -> (-123.9, 30.8932) centre (-123.9, 28.8932) ccw
  line L214 (-121.9, 28.8932) -> (-121.9, 20.3932)
  arc A226 (-104.9, 20.6932) -> (-102.9, 22.6932) centre (-104.9, 22.6932) ccw
  line L215 (-104.9, 20.6932) -> (-117.9, 20.6932)
  arc A227 (-119.9, 22.6932) -> (-117.9, 20.6932) centre (-117.9, 22.6932) ccw
  line L216 (-119.9, 22.6932) -> (-119.9, 30.7719)
  line L217 (-117.4787, 33.1932) -> (-104.9, 33.1932)
  arc A228 (-102.9, 31.1932) -> (-104.9, 33.1932) centre (-104.9, 31.1932) ccw
  line L218 (-102.9, 31.1932) -> (-102.9, 22.6932)
  arc A229 (-85.9, 28.6932) -> (-83.9, 30.6932) centre (-85.9, 30.6932) ccw
  line L219 (-85.9, 28.6932) -> (-98.9, 28.6932)
  arc A230 (-100.9, 30.6932) -> (-98.9, 28.6932) centre (-98.9, 30.6932) ccw
  line L220 (-100.9, 30.6932) -> (-100.9, 39.1932)
  arc A231 (-98.9, 41.1932) -> (-100.9, 39.1932) centre (-98.9, 39.1932) ccw
  line L221 (-98.9, 41.1932) -> (-85.9, 41.1932)
  arc A232 (-83.9, 39.1932) -> (-85.9, 41.1932) centre (-85.9, 39.1932) ccw
  line L222 (-83.9, 39.1932) -> (-83.9, 30.6932)
  arc A233 (-66.9, 32.1932) -> (-64.9, 34.1932) centre (-66.9, 34.1932) ccw
  line L223 (-66.9, 32.1932) -> (-79.9, 32.1932)
  arc A234 (-81.9, 34.1932) -> (-79.9, 32.1932) centre (-79.9, 34.1932) ccw
  line L224 (-81.9, 34.1932) -> (-81.9, 42.6932)
  arc A235 (-79.9, 44.6932) -> (-81.9, 42.6932) centre (-79.9, 42.6932) ccw
  line L225 (-79.9, 44.6932) -> (-66.9, 44.6932)
  arc A236 (-64.9, 42.6932) -> (-66.9, 44.6932) centre (-66.9, 42.6932) ccw
  line L226 (-64.9, 42.6932) -> (-64.9, 34.1932)
  arc A237 (-47.9, 27.6932) -> (-45.9, 29.6932) centre (-47.9, 29.6932) ccw
  line L227 (-47.9, 27.6932) -> (-60.9, 27.6932)
  arc A238 (-62.9, 29.6932) -> (-60.9, 27.6932) centre (-60.9, 29.6932) ccw
  line L228 (-62.9, 29.6932) -> (-62.9, 38.1932)
  arc A239 (-60.9, 40.1932) -> (-62.9, 38.1932) centre (-60.9, 38.1932) ccw
  line L229 (-60.9, 40.1932) -> (-47.9, 40.1932)
  arc A240 (-45.9, 38.1932) -> (-47.9, 40.1932) centre (-47.9, 38.1932) ccw
  line L230 (-45.9, 38.1932) -> (-45.9, 29.6932)
  arc A241 (-28.9, 25.3932) -> (-26.9, 27.3932) centre (-28.9, 27.3932) ccw
  line L231 (-28.9, 25.3932) -> (-41.9, 25.3932)
  arc A242 (-43.9, 27.3932) -> (-41.9, 25.3932) centre (-41.9, 27.3932) ccw
  line L232 (-43.9, 27.3932) -> (-43.9, 35.8932)
  arc A243 (-41.9, 37.8932) -> (-43.9, 35.8932) centre (-41.9, 35.8932) ccw
  line L233 (-41.9, 37.8932) -> (-28.9, 37.8932)
  arc A244 (-26.9, 35.8932) -> (-28.9, 37.8932) centre (-28.9, 35.8932) ccw
  line L234 (-26.9, 35.8932) -> (-26.9, 27.3932)
  arc A245 (-60.9, 21.1932) -> (-62.9, 19.1932) centre (-60.9, 19.1932) ccw
  line L235 (-62.9, 10.6932) -> (-62.9, 19.1932)
  arc A246 (-62.9, 10.6932) -> (-60.9, 8.6932) centre (-60.9, 10.6932) ccw
  line L236 (-47.9, 8.6932) -> (-60.9, 8.6932)
  arc A247 (-47.9, 8.6932) -> (-45.9, 10.6932) centre (-47.9, 10.6932) ccw
  line L237 (-28.9, 6.3932) -> (-41.9, 6.3932)
  arc A248 (-28.9, 6.3932) -> (-26.9, 8.3932) centre (-28.9, 8.3932) ccw
  line L238 (-26.9, 16.8932) -> (-26.9, 8.3932)
  arc A249 (-26.9, 16.8932) -> (-28.9, 18.8932) centre (-28.9, 16.8932) ccw
  line L239 (-41.9, 18.8932) -> (-28.9, 18.8932)
  arc A250 (-41.9, 18.8932) -> (-43.9, 16.8932) centre (-41.9, 16.8932) ccw
  line L240 (-43.9, 8.3932) -> (-43.9, 16.8932)
  arc A251 (-43.9, 8.3932) -> (-41.9, 6.3932) centre (-41.9, 8.3932) ccw
  arc A252 (-9.9, 4.0932) -> (-7.9, 6.0932) centre (-9.9, 6.0932) ccw
  line L241 (-9.9, 4.0932) -> (-22.9, 4.0932)
  arc A253 (-24.9, 6.0932) -> (-22.9, 4.0932) centre (-22.9, 6.0932) ccw
  line L242 (-24.9, 6.0932) -> (-24.9, 14.5932)
  arc A254 (-22.9, 16.5932) -> (-24.9, 14.5932) centre (-22.9, 14.5932) ccw
  line L243 (-22.9, 16.5932) -> (-9.9, 16.5932)
  arc A255 (-7.9, 14.5932) -> (-9.9, 16.5932) centre (-9.9, 14.5932) ccw
  line L244 (-7.9, 14.5932) -> (-7.9, 6.0932)
  line L245 (-60.9, 21.1932) -> (-48.3213, 21.1932)
  line L246 (-45.9, 18.7719) -> (-45.9, 10.6932)
  line L247 (-47.2607, 20.7539) -> (-46.3393, 19.8325)
  arc A256 (-47.2607, 20.7539) -> (-48.3213, 21.1932) centre (-48.3213, 19.6932) ccw
  arc A257 (-45.9, 18.7719) -> (-46.3393, 19.8325) centre (-47.4, 18.7719) ccw
  line L248 (-47.2607, 58.7539) -> (-46.3393, 57.8325)
  arc A258 (-47.2607, 58.7539) -> (-48.3213, 59.1932) centre (-48.3213, 57.6932) ccw
  arc A259 (-45.9, 56.7719) -> (-46.3393, 57.8325) centre (-47.4, 56.7719) ccw
  line L249 (-119.4607, 31.8325) -> (-118.5393, 32.7539)
  arc A260 (-119.4607, 31.8325) -> (-119.9, 30.7719) centre (-118.4, 30.7719) ccw
  arc A261 (-117.4787, 33.1932) -> (-118.5393, 32.7539) centre (-117.4787, 31.6932) ccw
  line L250 (-119.4607, 50.8325) -> (-118.5393, 51.7539)
  arc A262 (-117.4787, 52.1932) -> (-118.5393, 51.7539) centre (-117.4787, 50.6932) ccw
  arc A263 (-119.4607, 50.8325) -> (-119.9, 49.7719) centre (-118.4, 49.7719) ccw
  arc A264 (-7.6, 40.5932) -> (-7, 39.9932) centre (-7, 40.5932) ccw
  line L251 (-22.9, 75.8932) -> (-9.9, 75.8932)
  line L252 (-22.9, 37.8932) -> (-9.9, 37.8932)
  dimension "d1" = 3.4
  dimension "d2" = 3.4
  dimension "d3" = 8
  dimension "d4" = 3.4
  dimension "d5" = 3.4
  dimension "d9" = 2.2
  dimension "d12" = 2.2
  dimension "d318" = 4.2
  dimension "d319" = 4.2
  constraint tangent L19 A5
  constraint tangent L19 A6
  constraint tangent L13 A7
  constraint tangent L17 A8
  constraint tangent L12 A9
  constraint tangent L16 A10
  constraint tangent L8 A11
  constraint tangent L7 A13
  constraint tangent L9 A14
  constraint tangent L18 A15
  constraint tangent L2 A16
  constraint tangent L0 A17
  constraint tangent L10 A18
  constraint tangent L5 A19
  constraint tangent L11 A20
  constraint tangent L6 A21
  constraint tangent L3 A22
  constraint tangent L1 A23
  constraint tangent L4 A24
  constraint tangent A24 L104
  constraint perpendicular L104 L105
  constraint tangent L104 A25
  constraint tangent L105 A25
  constraint coincident L15.end L105
  constraint perpendicular L15 L105
  constraint coincident L14.end L104
  constraint perpendicular L14 L104
  constraint tangent L32 A26
  constraint tangent L33 A27
  constraint tangent L35 A28
  constraint tangent L34 A29
  constraint tangent L49 A30
  constraint tangent L49 A31
  constraint tangent L51 A32
  constraint tangent L50 A33
  constraint tangent L57 A34
  constraint tangent L57 A35
  constraint tangent L59 A36
  constraint tangent L58 A37
  constraint tangent L76 A38
  constraint tangent L78 A39
  constraint tangent L79 A40
  constraint tangent L77 A41
  constraint tangent L54 A42
  constraint tangent L54 A43
  constraint tangent L52 A44
  constraint tangent L53 A45
  constraint tangent L90 A46
  constraint tangent L90 A47
  constraint tangent L91 A47
  constraint tangent L91 A48
  constraint tangent L89 A49
  constraint tangent L100 A50
  constraint tangent L101 A51
  constraint tangent L103 A52
  constraint tangent L102 A53
  constraint tangent L93 A54
  constraint tangent L93 A55
  constraint tangent L95 A56
  constraint tangent L94 A57
  constraint tangent L21 A58
  constraint tangent L20 A59
  constraint tangent L22 A59
  constraint tangent L22 A60
  constraint tangent L23 A61
  constraint tangent L64 A62
  constraint tangent L66 A62
  constraint tangent L64 A63
  constraint tangent L65 A64
  constraint tangent L67 A65
  constraint tangent L98 A66
  constraint tangent L98 A67
  constraint tangent L96 A68
  constraint tangent L97 A69
  constraint tangent L70 A70
  constraint tangent L70 A71
  constraint tangent L68 A72
  constraint tangent L69 A73
  constraint tangent L80 A74
  constraint tangent L80 A75
  constraint tangent L82 A75
  constraint tangent L82 A76
  constraint tangent L83 A76
  constraint tangent L83 A77
  constraint tangent L81 A77
  constraint tangent L29 A78
  constraint tangent L29 A79
  constraint tangent L28 A80
  constraint tangent L30 A81
  constraint tangent L37 A82
  constraint tangent L37 A83
  constraint tangent L36 A83
  constraint tangent L36 A84
  constraint tangent L38 A84
  constraint tangent L38 A85
  constraint tangent L39 A85
  constraint tangent L61 A86
  constraint tangent L61 A87
  constraint tangent L60 A87
  constraint tangent L60 A88
  constraint tangent L62 A89
  constraint tangent L40 A90
  constraint tangent L42 A91
  constraint tangent L43 A92
  constraint tangent L41 A92
  constraint tangent L41 A93
  constraint tangent L40 A93
  constraint tangent L44 A94
  constraint tangent L46 A94
  constraint tangent L46 A95
  constraint tangent L47 A95
  constraint tangent L47 A96
  constraint tangent L45 A96
  constraint tangent L45 A97
  constraint tangent L44 A97
  constraint tangent L74 A98
  constraint tangent L75 A98
  constraint tangent L74 A99
  constraint tangent L72 A100
  constraint tangent L73 A101
  constraint tangent L26 A102
  constraint tangent L27 A102
  constraint tangent L26 A103
  constraint tangent L24 A104
  constraint tangent L25 A105
  constraint tangent L86 A106
  constraint tangent L87 A106
  constraint tangent L86 A107
  constraint tangent L84 A108
  constraint tangent L85 A109
  constraint tangent A12 L112
  constraint tangent L111 A112
  constraint tangent L112 A112
  constraint concentric A8 A113
  constraint concentric A6 A114
  constraint concentric A23 A115
  constraint concentric A21 A116
  constraint parallel L113 L136
  constraint tangent A117 L136
  constraint tangent L114 A117
  constraint tangent L113 A118
  constraint tangent L114 A118
  constraint horizontal L115
  constraint perpendicular L115 L116
  constraint parallel L115 L117
  constraint parallel L116 L118
  constraint tangent A120 L118
  constraint tangent L117 A120
  constraint tangent L116 A119
  constraint tangent A119 L117
  constraint horizontal L119
  constraint perpendicular L119 L120
  constraint parallel L119 L121
  constraint parallel L120 L122
  constraint tangent A122 L122
  constraint tangent L121 A122
  constraint tangent L120 A121
  constraint tangent A121 L121
  constraint horizontal L123
  constraint perpendicular L123 L124
  constraint parallel L123 L125
  constraint parallel L124 L126
  constraint tangent A124 L126
  constraint tangent L125 A124
  constraint tangent L124 A123
  constraint tangent A123 L125
  constraint horizontal L127
  constraint perpendicular L127 L128
  constraint parallel L127 L129
  constraint parallel L128 L130
  constraint tangent A126 L130
  constraint tangent L129 A126
  constraint tangent L128 A125
  constraint tangent A125 L129
  constraint horizontal L135
  constraint perpendicular L131 L135
  constraint parallel L132 L135
  constraint parallel L131 L133
  constraint tangent A128 L133
  constraint tangent L132 A128
  constraint tangent L131 A127
  constraint tangent A127 L132
  constraint horizontal L134
  constraint perpendicular L134 L176
  constraint parallel L176 L178
  constraint tangent A132 L178
  constraint tangent A129 L134
  constraint tangent A129 L178
  constraint tangent L134 A130
  constraint tangent A130 L176
  constraint tangent A131 L176
  constraint coincident L164 L107.end
  constraint coincident L165 L106.end
  constraint tangent L171 A155
  constraint tangent L172 A155
  constraint tangent L171 A156
  constraint tangent L170 A156
  constraint tangent L166 A157
  constraint tangent L165 A157
  constraint tangent L164 A158
  constraint tangent L165 A158
  constraint tangent L160 A159
  constraint tangent L168 A160
  constraint tangent L173 A160
  constraint tangent L169 A161
  constraint tangent L173 A161
  constraint tangent L169 A162
  constraint tangent L174 A162
  constraint tangent L170 A163
  constraint tangent L174 A163
  constraint coincident L147 L107.start
  constraint coincident L148 L106.start
  constraint perpendicular L165 L175
  constraint collinear L176 L177
  constraint collinear L178 L179
  constraint tangent L177 A164
  constraint tangent L178 A165
  constraint tangent L175 A166
  constraint tangent L176 A166
  constraint tangent L175 A167
  constraint tangent L179 A167
  constraint tangent A159 L181
  constraint tangent L168 A168
  constraint tangent L186 A168
  constraint tangent L167 A169
  constraint tangent L185 A169
  constraint tangent L167 A170
  constraint tangent L186 A170
  constraint tangent L166 A171
  constraint tangent L185 A171
  constraint tangent L164 A172
  constraint tangent L184 A172
  constraint tangent L163 A173
  constraint tangent L184 A173
  constraint tangent L162 A174
  constraint tangent L182 A174
  constraint tangent L162 A175
  constraint tangent L183 A175
  constraint tangent L163 A176
  constraint tangent L183 A176
  constraint tangent L161 A177
  constraint tangent L182 A177
  constraint tangent L161 A178
  constraint tangent L181 A178
  constraint tangent L160 A179
  constraint tangent L180 A179
  constraint tangent L172 A180
  constraint tangent L180 A180
  constraint concentric A110 A181
  constraint concentric A111 A182
  constraint tangent L110 A183
  constraint tangent L110 A184
  constraint tangent L108 A185
  constraint tangent L108 A186
  constraint tangent L109 A186
  constraint tangent L15 A187
  constraint tangent L14 A187
  constraint tangent L137 A188
  constraint tangent L113 A188
  constraint tangent L136 A189
  constraint tangent L137 A189
  constraint tangent L116 A190
  constraint tangent L115 A190
  constraint tangent L118 A191
  constraint tangent L115 A191
  constraint tangent L120 A192
  constraint tangent L119 A192
  constraint tangent L122 A193
  constraint tangent L119 A193
  constraint tangent L124 A194
  constraint tangent L123 A194
  constraint tangent L126 A195
  constraint tangent L123 A195
  constraint tangent L128 A196
  constraint tangent L127 A196
  constraint tangent L130 A197
  constraint tangent L127 A197
  constraint tangent L131 A198
  constraint tangent L135 A198
  constraint tangent L135 A199
  constraint tangent L133 A199
  constraint parallel L187 L189
  constraint tangent L187 A200
  constraint tangent A200 L188
  constraint tangent A201 L189
  constraint tangent L188 A201
  constraint horizontal L191
  constraint perpendicular L191 L192
  constraint parallel L191 L193
  constraint parallel L192 L194
  constraint tangent A206 L194
  constraint tangent L193 A206
  constraint horizontal L195
  constraint perpendicular L195 L196
  constraint parallel L195 L197
  constraint parallel L196 L198
  constraint tangent A210 L198
  constraint tangent L197 A210
  constraint tangent L196 A209
  constraint tangent A209 L197
  constraint horizontal L201
  constraint perpendicular L201 L202
  constraint parallel L199 L201
  constraint parallel L200 L202
  constraint tangent A212 L200
  constraint tangent L199 A212
  constraint tangent A211 L202
  constraint tangent A211 L199
  constraint horizontal L205
  constraint perpendicular L205 L206 L39
  constraint parallel L203 L205
  constraint parallel L204 L206 L39
  constraint tangent A215 L206 L39
  constraint tangent A215 L203
  constraint horizontal L209
  constraint perpendicular L209 L210
  constraint parallel L207 L209
  constraint parallel L208 L210
  constraint tangent A219 L208
  constraint tangent L207 A219
  constraint tangent A218 L210
  constraint tangent A218 L207
  constraint tangent A202 L190
  constraint tangent L189 A202
  constraint tangent L187 A203
  constraint tangent L190 A203
  constraint tangent A205 L192
  constraint tangent L191 A205
  constraint tangent A204 L194
  constraint tangent A204 L191
  constraint tangent A208 L196
  constraint tangent L195 A208
  constraint tangent A207 L198
  constraint tangent A207 L195
  constraint tangent A214 L202
  constraint tangent L201 A214
  constraint tangent L200 A213
  constraint tangent A213 L201
  constraint tangent A217 L206 L39
  constraint tangent L205 A217
  constraint tangent L204 A216
  constraint tangent A216 L205
  constraint tangent A221 L210
  constraint tangent L209 A221
  constraint tangent A220 L209
  constraint tangent L208 A220
  constraint parallel L212 L214
  constraint tangent A225 L214
  constraint tangent L213 A225
  constraint tangent L212 A224
  constraint tangent A224 L213
  constraint horizontal L215
  constraint perpendicular L215 L216
  constraint parallel L215 L217
  constraint parallel L216 L218
  constraint tangent A228 L218
  constraint tangent L217 A228
  constraint horizontal L219
  constraint perpendicular L219 L220
  constraint parallel L219 L221
  constraint parallel L220 L222
  constraint tangent A232 L222
  constraint tangent L221 A232
  constraint tangent L220 A231
  constraint tangent A231 L221
  constraint horizontal L223
  constraint perpendicular L223 L224
  constraint parallel L223 L225
  constraint parallel L224 L226
  constraint tangent A236 L226
  constraint tangent L225 A236
  constraint tangent L224 A235 L40.start
  constraint tangent A235 L40.start L225
  constraint horizontal L227
  constraint perpendicular L227 L228
  constraint parallel L227 L229
  constraint parallel L228 L230
  constraint tangent A240 L230
  constraint tangent L229 A240
  constraint tangent L228 A239
  constraint tangent A239 L229
  constraint horizontal L231
  constraint perpendicular L231 L232
  constraint parallel L231 L233
  constraint parallel L232 L234
  constraint tangent A244 L234
  constraint tangent L233 A244
  constraint tangent L232 A243
  constraint tangent A243 L233
  constraint tangent L211 A223
  constraint tangent A223 L212
  constraint tangent A222 L214
  constraint tangent A222 L211
  constraint tangent A227 L216
  constraint tangent L215 A227
  constraint tangent A226 L218
  constraint tangent A226 L215
  constraint tangent A230 L220
  constraint tangent L219 A230
  constraint tangent A229 L222
  constraint tangent A229 L219
  constraint tangent A234 L224
  constraint tangent L223 A234
  constraint tangent A233 L226
  constraint tangent A233 L223
  constraint tangent A238 L228
  constraint tangent L227 A238
  constraint tangent A237 L230
  constraint tangent A237 L227
  constraint tangent A242 L232
  constraint tangent L231 A242
  constraint tangent A241 L231
  constraint tangent A241 L234
  constraint horizontal L236
  constraint perpendicular L235 L236
  constraint parallel L236 L245
  constraint tangent A245 L235
  constraint tangent A245 L245
  constraint horizontal L237
  constraint perpendicular L237 L240
  constraint parallel L237 L239
  constraint parallel L238 L240
  constraint tangent L238 A249
  constraint tangent A249 L239
  constraint tangent A250 L240
  constraint tangent L239 A250
  constraint tangent L235 A246
  constraint tangent A246 L236
  constraint tangent L236 A247
  constraint tangent L240 A251
  constraint tangent L237 A251
  constraint tangent L237 A248
  constraint tangent A248 L238
  constraint horizontal L241
  constraint perpendicular L241 L242
  constraint parallel L241 L243
  constraint parallel L242 L244
  constraint tangent A255 L244
  constraint tangent L243 A255
  constraint tangent L242 A254